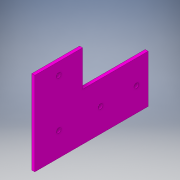
# Autodesk Inventor part: Inside L Plate
Saved by Autodesk Inventor 2017 (Build 210142000, 142)
## iProperties
Created: 2017-01-21
Part Number: Inside L Plate
Material: Generic
Document SubType Name: Modeling
Designer: Ben
Density: 1 g/cm^3
Appearance: Magenta
Author: Ben
Autodesk Inventor part; units mm, degrees
ref_plane "YZ Plane" through (0, 0, 0) normal (1, 0, 0) x (0, 1, 0)
ref_plane "XZ Plane" through (0, 0, 0) normal (0, 1, 0) x (-1, 0, 0)
ref_plane "XY Plane" through (0, 0, 0) normal (0, 0, 1) x (1, 0, 0)
sketch "Sketch1" plane through (0, 0, 0) normal (1, 0, 0) x (0, 1, 0)
  circle A0 centre (0, 0) radius 1.27
  line L0 (0, 0) -> (25.4, 0) construction
  line L1 (0, 0) -> (0, -41.275) construction
  circle A1 centre (25.4, 0) radius 1.27
  circle A2 centre (0, -22.225) radius 1.27
  circle A3 centre (0, -41.275) radius 1.27
  line L2 (31.75, 12.7) -> (31.75, -12.7)
  line L3 (31.75, -12.7) -> (12.7, -12.7)
  line L4 (12.7, -12.7) -> (12.7, -47.625)
  line L5 (12.7, -47.625) -> (-12.7, -47.625)
  line L6 (-12.7, -47.625) -> (-12.7, 12.7)
  line L7 (-12.7, 12.7) -> (31.75, 12.7)
  line L8 (25.4, 0) -> (31.75, 0) construction
  line L9 (0, -41.275) -> (0, -47.625) construction
  dimension "d0" = 2.54
  dimension "d1" = 25.4
  dimension "d2" = 22.225
  dimension "d3" = 19.05
  dimension "d4" = 25.4
  dimension "d5" = 6.35
  dimension "d6" = 6.35
  constraints: 20 end point, 6 perpendicular, 4 centre point, 3 coincident, 3 equal radius, 3 vertical, 2 horizontal, 2 midpoint, 1 point on line
  measures "d0" diameter of A0
  measures "d1" distance of L0.end point (0, 0)
  measures "d2" distance of A2.centre point (0, 0)
  measures "d3" distance of A2.centre L1.end
  measures "d4" distance of L4.end L5.end
  measures "d5" distance from line of L1.end L5
  measures "d6" distance from line of L2 L0.end
extrude "Extrusion1" add sketch "Sketch1" along normal blind 1.5875
equation "\"d6\" = d5"
body "Solid1"
